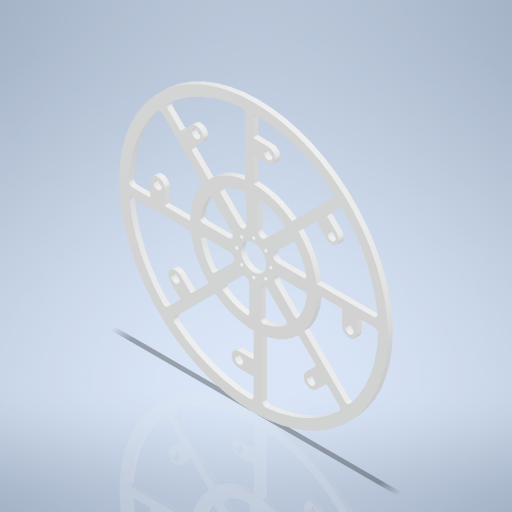
# Autodesk Inventor part: 211
Saved by Autodesk Inventor 2024 (Build 280153000, 153)
## iProperties
Created: 2024-06-10
Part Number: 211
Material: Aluminium 6061
Document SubType Name: Modeling
Designer: ffogue
Density: 2.7 g/cm^3
Appearance: Aluminium - flach
Author: ffogue
Autodesk Inventor part; units mm, degrees
ref_plane "YZ Plane" through (0, 0, 0) normal (1, 0, 0) x (0, 1, 0)
ref_plane "XZ Plane" through (0, 0, 0) normal (0, 1, 0) x (-1, 0, 0)
ref_plane "XY Plane" through (0, 0, 0) normal (0, 0, 1) x (1, 0, 0)
sketch "Skizze1" plane through (0, 0, 0) normal (0, 1, 0) x (-1, 0, 0)
  circle A0 centre (0, 0) radius 110
  dimension "d0" = 220
  constraints: 1 centre point, 1 coincident
  measures "d0" diameter of A0
extrude "Extrusion1" add sketch "Skizze1" along normal blind 4
sketch "Skizze2" plane through (0, 0, 0) normal (0, -1, 0) x (1, 0, 0)
  arc A0 (-7, 101.7595) -> (-72.1249, 72.1249) centre (0, 0) ccw
  circle A1 centre (0, 0) radius 110 projected
  line L0 (-7, 51.5267) -> (-7, 101.7595)
  arc A2 (-7, 51.5267) -> (-36.7696, 36.7696) centre (0, 0) ccw
  line L1 (-36.7696, 36.7696) -> (-72.1249, 72.1249)
  line L2 (0, 0) -> (-110, 0) construction
  dimension "d4" = 7
  dimension "d6" = 45
  dimension "d9" = 8
  dimension "d10" = 50
  dimension "d11" = 50
  constraints: 6 end point, 4 point on circle, 2 centre point, 1 coincident, 1 horizontal, 1 horizontal alignment, 1 vertical, 2 other
  measures "d4" distance from line of point (0, 0) L0
  measures "d6" angle of L2 L1
  measures "d10" radial gap between concentric circles of A2 A0
  measures "d11" distance of L1.start L1.end
extrude "Extrusion2" cut sketch "Skizze2" against normal up to surface (4 mm away) contours L0 A2 L1 A0
pattern_circular "Runde Anordnung1" count 8 over 360 about axis through (0, 0, 0) along (0, 1, 0) of "Extrusion2"
sketch "Skizze3" plane through (0, 0, 0) normal (0, -1, 0) x (1, 0, 0)
  circle A0 centre (0, 0) radius 10.5
  dimension "d17" = 21
  constraints: 1 centre point, 1 coincident
  measures "d17" diameter of A0
extrude "Extrusion3" cut sketch "Skizze3" against normal up to surface (4 mm away)
sketch "Skizze5" plane through (0, 0, 0) normal (0, -1, 0) x (1, 0, 0)
  circle A0 centre (0, 0) radius 14 construction
  point P0 (0, 14)
  dimension "d20" = 28
  constraints: 2 vertical alignment, 1 coincident, 2 other
hole "Bohrung1" at (0, 0, 14) direction (0, 1, 0) diameter 3 end through all
pattern_circular "Runde Anordnung2" count 8 over 360 about axis through (0, 0, 0) along (0, 1, 0) of "Bohrung1"
sketch "Skizze6" plane through (0, 0, 0) normal (0, -1, 0) x (1, 0, 0)
  circle A0 centre (0, 0) radius 21.5 construction
  arc A1 (-35.0188, 26.6399) -> (-43.8606, 3.5) centre (0, 0) ccw
  arc A2 (-7, 51.5267) -> (-36.7696, 36.7696) centre (0, 0) ccw projected
  line L0 (-35.0188, 26.6399) -> (-17.8537, 9.4749)
  line L1 (0, 0) -> (0, 61.7697) construction
  line L2 (0, 52) -> (0, 102) projected
  line L3 (-43.8606, 3.5) -> (-20.3286, 3.5)
  arc A3 (-20.3286, 3.5) -> (-17.8537, 9.4749) centre (-20.3286, 7) ccw
  line L4 (-76.9046, 67.0051) -> (-41.3846, 31.4851) projected
  line L5 (-7, 101.7595) -> (-7, 51.5267) projected
  line L6 (-36.7696, 36.7696) -> (-72.1249, 72.1249) projected
  dimension "d31" = 43
  dimension "d33" = 44
  dimension "d34" = 3.5
  dimension "d35" = 3.5
  constraints: 6 end point, 4 point on circle, 2 centre point, 2 parallel, 2 tangent, 1 coincident, 1 concentric, 1 point on line, 3 other
  measures "d33" radius of A1
  measures "d34" distance from line of point (0, 0) L3
  measures "d35" radius of A3
extrude "Extrusion4" cut sketch "Skizze6" against normal up to surface (4 mm away)
fillet "Rundung1" radius 2 2 edges at (-43.8606, 2, 3.5) (-35.0188, 2, 26.6399)
pattern_circular "Runde Anordnung3" count 8 over 360 about axis through (0, 0, 0) along (0, 1, 0) of "Extrusion4", "Rundung1"
fillet "Rundung2" radius 3 2 edges at (0, 2, -102) (-67.0051, 2, -76.9046)
pattern_circular "Runde Anordnung4" count 8 over 360 about axis through (0, 0, 0) along (0, 1, 0) of "Rundung2"
sketch "Skizze7" plane through (0, 0, 0) normal (0, -1, 0) x (1, 0, 0)
  line L0 (0, 98.9545) -> (0, 52) projected
  line L1 (0, 84.5) -> (12, 84.5)
  arc A0 (12, 72.5) -> (12, 84.5) centre (12, 78.5) ccw
  line L2 (12, 72.5) -> (0, 72.5)
  circle A1 centre (12, 78.5) radius 3.5
  point P0 (0, 0)
  dimension "d46" = 6
  dimension "d47" = 78.5
  dimension "d48" = 12
  dimension "d49" = 7
  constraints: 4 end point, 2 centre point, 2 point on circle, 2 point on line, 2 tangent, 1 coincident, 1 horizontal, 1 parallel
  measures "d46" radius of A0
  measures "d47" vertical distance of point (0, 0) A0.centre
  measures "d48" distance from line of L0 A0.centre
  measures "d49" diameter of A1
extrude "Extrusion5" add sketch "Skizze7" against normal up to surface (4 mm away)
fillet "Rundung3" radius 1 2 edges at (0, 2, 72.5) (0, 2, 84.5)
pattern_circular "Runde Anordnung5" count 8 over 360 about axis through (0, 0, 0) along (0, 1, 0) of "Extrusion5", "Rundung3"
